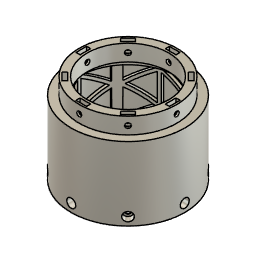
section_fuselage_30mm_ISO v15 (Autodesk Fusion 360 design; units mm, degrees)
Autodesk Fusion 360 part; units mm, degrees
note: some values were not read from the file. Set by a fixed rule: which face or edge a step refers to.
sketch "Esquisse1" plane through (0, 0, 0) normal (0, 1, 0) x (1, 0, 0)
  circle A0 centre (0, 0) radius 35
  circle A1 centre (0, 0) radius 30
  dimension "d1" = 70
  dimension "d2" = 60
  constraint coincident A0.centre A1.centre
  measures "d1" diameter of A0
  measures "d2" diameter of A1
extrude "Extrusion1" add sketch "Esquisse1" along normal mid plane 150 makes body 1
ref_plane "Plan de construction1" through (-30, 0, 0) normal (1, 0, 0) x (0, 1, 0)
sketch "Esquisse2" plane through (-30, 0, 0) normal (1, 0, 0) x (0, 0, -1)
  line L0 (-10, 75) -> (10, 75) construction
  line L1 (10, -75) -> (-10, -75) construction
  line L2 (0, 75) -> (0, -75) construction
  line L3 (0, 75) -> (0, 55) construction
  line L4 (0, 55) -> (0, 75) construction
  line L5 (0, 75) -> (17.3205, 65) construction
  line L6 (17.3205, 65) -> (0, 55) construction
  line L7 (0, 75) -> (-0.866, 75.5) construction
  line L8 (0, 75) -> (0, 76) construction
  line L9 (0.6, 54.2) -> (17.8202, 64.1338)
  line L10 (-0.494, 74.1306) -> (0, 75) construction
  line L11 (0, 75) -> (0.5, 75.866) construction
  line L12 (0.5, 75.866) -> (17.8205, 65.866)
  line L13 (15.4471, 65.0724) -> (1, 73.2816)
  line L14 (0, 73.8498) -> (-0.494, 74.1306)
  line L15 (1, 74.4227) -> (1, 75)
  line L16 (16.3207, 65.5772) -> (16.8202, 65.8658)
  line L17 (1, 56.7245) -> (1, 73.2816)
  line L18 (1, 56.7245) -> (15.4471, 65.0724)
  line L19 (-1, 56.7245) -> (-15.4471, 65.0724)
  line L20 (-1, 56.7245) -> (-1, 73.2816)
  line L21 (-15.4471, 65.0724) -> (-1, 73.2816)
  line L22 (-17.3205, 65) -> (0, 75) construction
  line L23 (0, 55) -> (-17.3205, 65) construction
  line L24 (-1, 74.4227) -> (-1, 75)
  line L25 (-1, 56.7245) -> (-1, 73.2816)
  line L26 (-16.3211, 66.5862) -> (-1.9882, 74.9932)
  line L27 (-16.327, 83.2717) -> (-16.3211, 66.5862)
  line L28 (-16.327, 83.2717) -> (-1.9882, 74.9932)
  circle A0 centre (-17.3205, 85) radius 1
  line L29 (16.327, 83.2717) -> (1.9882, 74.9932)
  line L30 (16.3211, 66.5862) -> (1.9882, 74.9932)
  line L31 (16.327, 83.2717) -> (16.3211, 66.5862)
  circle A1 centre (17.3205, 85) radius 1
  line L32 (-20.0336, 74.9932) -> (20, 74.9932)
  line L33 (0, 55) -> (-5, 55) construction
  line L34 (-1.9935, 55.0038) -> (-16.4465, 63.3414)
  line L35 (-16.4465, 63.3414) -> (-16.3323, 46.7252)
  line L36 (-1.9935, 55.0038) -> (-16.3323, 46.7252)
  line L37 (-0.9935, 53.2717) -> (-0.9994, 36.5862)
  line L38 (-0.9935, 53.2717) -> (-15.3323, 44.9932)
  line L39 (-0.9994, 36.5862) -> (-15.3323, 44.9932)
  line L40 (1.9935, 55.0038) -> (16.4465, 63.3414)
  line L41 (1.9935, 55.0038) -> (16.3323, 46.7252)
  line L42 (16.4465, 63.3414) -> (16.3323, 46.7252)
  line L43 (0.9935, 53.2717) -> (15.3323, 44.9932)
  line L44 (0.9994, 36.5862) -> (15.3323, 44.9932)
  line L45 (0.9935, 53.2717) -> (0.9994, 36.5862)
  line L46 (0, 35) -> (-15, 35) construction
  line L47 (-16.4465, 6.6586) -> (-16.3323, 23.2748)
  line L48 (-1.9935, 14.9962) -> (-16.4465, 6.6586)
  line L49 (-1, 13.2755) -> (-15.4471, 4.9276)
  line L50 (-15.4471, 4.9276) -> (-1, -3.2816)
  line L51 (-1, 13.2755) -> (-1, -3.2816)
  line L52 (15.4471, 4.9276) -> (1, -3.2816)
  line L53 (1, 13.2755) -> (1, -3.2816)
  line L54 (1, 13.2755) -> (15.4471, 4.9276)
  line L55 (1.9935, 14.9962) -> (16.4465, 6.6586)
  line L56 (16.4465, 6.6586) -> (16.3323, 23.2748)
  line L57 (1.9935, 14.9962) -> (16.3323, 23.2748)
  line L58 (0.9994, 33.4138) -> (15.3323, 25.0068)
  line L59 (0.9935, 16.7283) -> (15.3323, 25.0068)
  line L60 (0.9935, 16.7283) -> (0.9994, 33.4138)
  line L61 (-0.9994, 33.4138) -> (-15.3323, 25.0068)
  line L62 (-0.9935, 16.7283) -> (-15.3323, 25.0068)
  line L63 (-1.9935, 14.9962) -> (-16.3323, 23.2748)
  line L64 (-0.9935, 16.7283) -> (-0.9994, 33.4138)
  line L65 (0, -5) -> (-10, -5) construction
  line L66 (-1.8734, 35.0724) -> (-16.3205, 43.2816)
  line L67 (-16.3205, 26.7245) -> (-16.3205, 43.2816)
  line L68 (-16.3205, 26.7245) -> (-1.8734, 35.0724)
  line L69 (0, 35) -> (17.3205, 45) construction
  line L70 (1.8734, 35.0724) -> (16.3205, 43.2816)
  line L71 (16.3205, 26.7245) -> (16.3205, 43.2816)
  line L72 (16.3205, 26.7245) -> (1.8734, 35.0724)
  line L73 (0, -5) -> (-10, -5) construction
  line L74 (-15.4471, -14.9276) -> (-1, -6.7184)
  line L75 (-1, -23.2755) -> (-15.4471, -14.9276)
  line L76 (-1.9935, -24.9962) -> (-16.4465, -16.6586)
  line L77 (-1.9935, -24.9962) -> (-16.3323, -33.2748)
  line L78 (-16.4465, -16.6586) -> (-16.3323, -33.2748)
  line L79 (-0.9994, -43.4138) -> (-15.3323, -35.0068)
  line L80 (-0.9935, -26.7283) -> (-15.3323, -35.0068)
  line L81 (0.9935, -26.7283) -> (15.3323, -35.0068)
  line L82 (0.9994, -43.4138) -> (15.3323, -35.0068)
  line L83 (0.9935, -26.7283) -> (0.9994, -43.4138)
  line L84 (-0.9935, -26.7283) -> (-0.9994, -43.4138)
  line L85 (1.9935, -24.9962) -> (16.3323, -33.2748)
  line L86 (16.4465, -16.6586) -> (16.3323, -33.2748)
  line L87 (1.9935, -24.9962) -> (16.4465, -16.6586)
  line L88 (1, -23.2755) -> (15.4471, -14.9276)
  line L89 (1, -23.2755) -> (1, -6.7184)
  line L90 (-1, -23.2755) -> (-1, -6.7184)
  line L91 (15.4471, -14.9276) -> (1, -6.7184)
  line L92 (0, -45) -> (-15, -45) construction
  line L93 (-1.9935, -65.0038) -> (-16.3323, -56.7252)
  line L94 (1.9935, -65.0038) -> (16.3323, -56.7252)
  line L95 (-1, -66.7245) -> (-15.4471, -75.0724)
  circle A2 centre (0, -85) radius 1
  line L96 (0.9935, -63.2717) -> (15.3323, -54.9932)
  line L97 (0, -45) -> (-15, -45) construction
  line L98 (-0.9935, -63.2717) -> (-0.9994, -46.5862)
  line L99 (-0.9994, -46.5862) -> (-15.3323, -54.9932)
  line L100 (-16.4465, -73.3414) -> (-16.3323, -56.7252)
  line L101 (-1.9935, -65.0038) -> (-16.4465, -73.3414)
  line L102 (-0.9935, -63.2717) -> (-15.3323, -54.9932)
  line L103 (0.9994, -46.5862) -> (15.3323, -54.9932)
  circle A3 centre (0, -85) radius 1
  line L104 (0, -85) -> (-10, -85) construction
  line L105 (1, -66.7245) -> (15.4471, -75.0724)
  line L106 (-1, -66.7245) -> (-1, -83.2816)
  line L107 (0, -85) -> (-10, -85) construction
  line L108 (-15.4471, -75.0724) -> (-1, -83.2816)
  line L109 (16.4465, -73.3414) -> (16.3323, -56.7252)
  line L110 (1.9935, -65.0038) -> (16.4465, -73.3414)
  line L111 (15.4471, -75.0724) -> (1, -83.2816)
  line L112 (1, -66.7245) -> (1, -83.2816)
  line L113 (0.9935, -63.2717) -> (0.9994, -46.5862)
  line L114 (-20, -75) -> (25, -75)
  line L115 (-17.3205, 5) -> (0, -5) construction
  line L116 (0, -5) -> (17.3205, 5) construction
  line L117 (-17.3205, -35) -> (0, -45) construction
  line L118 (0, -45) -> (17.3205, -35) construction
  line L119 (-1.8734, -44.9276) -> (-16.3205, -36.7184)
  line L120 (-16.3205, -53.2755) -> (-16.3205, -36.7184)
  line L121 (-16.3205, -53.2755) -> (-1.8734, -44.9276)
  line L122 (16.3205, -53.2755) -> (1.8734, -44.9276)
  line L123 (16.3205, -53.2755) -> (16.3205, -36.7184)
  line L124 (1.8734, -44.9276) -> (16.3205, -36.7184)
  line L125 (-16.3211, 3.4138) -> (-1.9882, -4.9932)
  line L126 (-16.327, -13.2717) -> (-16.3211, 3.4138)
  line L127 (-16.327, -13.2717) -> (-1.9882, -4.9932)
  line L128 (16.327, -13.2717) -> (1.9882, -4.9932)
  line L129 (16.327, -13.2717) -> (16.3211, 3.4138)
  line L130 (16.3211, 3.4138) -> (1.9882, -4.9932)
  point P0 (0, -25)
  point P1 (0, -65)
  dimension "d7" = 20
  dimension "d9" = 20
  dimension "d10" = 60
  constraint horizontal L0
  constraint parallel L0 L1
  constraint midpoint L0 L2.start
  constraint midpoint L1 L2.end
  constraint perpendicular L1 L2
  constraint coincident L2 L3.end
  constraint coincident L0 L15.end
  constraint parallel L4 L8
  constraint perpendicular L7 L11
  constraint coincident L2 L14.start
  constraint collinear L13 L14
  constraint coincident L5 L15.start
  constraint coincident L5 L16.start
  constraint symmetric L3 L13.end L20.end
  constraint symmetric L3 L13.start L19.end
  constraint symmetric L3 L17.start L19.start
  constraint coincident L22 L24.start
  constraint symmetric L19.start L22 L27.start
  constraint symmetric L19.end L22 L26.start
  constraint symmetric L20.end L22 L26.end
  constraint symmetric L5 L13.end L29.end
  constraint symmetric L5 L13.start L30.start
  constraint symmetric L5 L17.start L29.start
  constraint parallel L0 L32
  constraint symmetric L13.end L23 L38.end
  constraint symmetric L13.start L23 L37.end
  constraint symmetric L17.start L23 L37.start
  constraint symmetric L19.start L23 L34.start
  constraint symmetric L19.end L23 L34.end
  constraint symmetric L20.end L23 L35.end
  constraint symmetric L6 L13.end L41.end
  constraint symmetric L6 L13.start L40.end
  constraint symmetric L6 L17.start L40.start
  constraint symmetric L2 L37.start L43.start
  constraint symmetric L2 L37.end L44.start
  constraint symmetric L2 L38.end L43.end
  constraint perpendicular L2 L46
  constraint symmetric L13.end L46 L52.end
  constraint symmetric L13.start L46 L52.start
  constraint symmetric L17.start L46 L53.start
  constraint symmetric L19.start L46 L49.start
  constraint symmetric L19.end L46 L49.end
  constraint symmetric L20.end L46 L50.end
  constraint symmetric L37.end L46 L61.start
  constraint symmetric L44.start L46 L58.start
  constraint symmetric L43.start L69 L71.start
  constraint symmetric L43.end L69 L70.end
  constraint symmetric L44.start L69 L70.start
  constraint symmetric L47.start L65 L76.end
  constraint symmetric L47.end L65 L77.end
  constraint symmetric L48.start L65 L76.start
  constraint symmetric L49.start L65 L75.start
  constraint symmetric L49.end L65 L74.start
  constraint symmetric L50.end L65 L74.end
  constraint symmetric L52.start L65 L88.end
  constraint symmetric L52.end L65 L89.end
  constraint symmetric L53.start L65 L88.start
  constraint symmetric L55.start L65 L85.start
  constraint symmetric L55.end L65 L86.start
  constraint symmetric L56.end L65 L85.end
  constraint symmetric L58.start L65 L82.start
  constraint symmetric L58.end L65 L81.end
  constraint symmetric L59.start L65 L81.start
  constraint symmetric L61.start L65 L79.start
  constraint symmetric L61.end L65 L79.end
  constraint symmetric L62.start L65 L80.start
  constraint symmetric L73.end L65 L65.end
  constraint symmetric L65.end L92 L104.end
  constraint symmetric P0 L92 P1
  constraint symmetric L74.start L92 L95.end
  constraint symmetric L74.end L92 L106.end
  constraint symmetric L75.start L92 L95.start
  constraint symmetric L76.start L92 L93.start
  constraint symmetric L76.end L92 L100.start
  constraint symmetric L77.end L92 L93.end
  constraint symmetric L79.start L92 L98.end
  constraint symmetric L79.end L92 L99.end
  constraint symmetric L80.start L92 L98.start
  constraint symmetric L81.start L92 L96.start
  constraint symmetric L81.end L92 L96.end
  constraint symmetric L82.start L92 L103.start
  constraint symmetric L85.start L92 L94.start
  constraint symmetric L85.end L92 L94.end
  constraint symmetric L86.start L92 L109.start
  constraint symmetric L88.start L92 L105.start
  constraint symmetric L88.end L92 L105.end
  constraint symmetric L89.end L92 L111.end
  constraint symmetric L97.start L92 L117.end
  constraint symmetric L97.end L92 L92.end
  constraint perpendicular L106 L114
  constraint symmetric L79.start L117 L119.start
  constraint symmetric L79.end L117 L119.end
  constraint symmetric L80.start L117 L120.start
  constraint symmetric L81.start L118 L122.start
  constraint symmetric L81.end L118 L123.end
  constraint symmetric L82.start L118 L122.end
  constraint symmetric L49.start L115 L126.start
  constraint symmetric L49.end L115 L125.start
  constraint symmetric L50.end L115 L125.end
  constraint symmetric L52.start L116 L129.end
  constraint symmetric L52.end L116 L128.end
  constraint symmetric L53.start L116 L128.start
  measures "d7" distance of L2.start L3.end
  measures "d9" distance of L2.start L5.end
  measures "d10" angle of L4 L5
emboss "Gravure en relief1" depth -2 profiles "Esquisse2" section 1 contours L9 L40 L41 L42 | L12 L31 L32 | L12 L30 L31 L32 | L13 L17 L18 | L19 L20 L21 L25 | L26 L27 L32 | L34 L35 L36 | L37 L38 L39 | L43 L44 L45 | L47 L48 L63 | L49 L50 L51 | L52 L53 L54 | L55 L56 L57 | L58 L59 L60 | L61 L62 L64 | L66 L67 L68 | L70 L71 L72 | L74 L75 L90 | L76 L77 L78 | L79 L80 L84 | L81 L82 L83 | L85 L86 L87 | L88 L89 L91 | L93 L100 L101 | L94 L109 L110 | L95 L106 L114 | L96 L103 L113 | L98 L99 L102 | L105 L112 L114 | L119 L120 L121 | L122 L123 L124 | L125 L126 L127 | L128 L129 L130 onto face at (29.9627, 50, 1.4954) on bodies 1 bodies 1
pattern_circular "Réseau C1" count 5 over 360 about axis through (0, 1.75, 0) along (0, 1, 0) of "Gravure en relief1"
extrude "Extrusion2" cut 1 faces at (33.0913, 75, 3.2292) along direction (0, -1, 0) blind 120 on bodies 1 bodies 1
sketch "Esquisse1 (2)" plane through (0, 0, 0) normal (0, 1, 0) x (1, 0, 0) in component "couplage_standard_femelle v11"
  circle A0 centre (0, 0) radius 35
  circle A1 centre (0, 0) radius 30
  dimension "d1_1" = 70
  dimension "d2_1" = 60
  constraint coincident A0.centre A1.centre
  constraint concentric A0 A1
  measures "d1_1" diameter of A0
  measures "d2_1" diameter of A1
extrude "Extrusion1'" add sketch "Esquisse1 (2)" along normal mid plane 10 separate body makes body 2 in component "couplage_standard_femelle v11"
ref_plane "Plan de construction1" through (35, 0, 0) normal (1, 0, 0) x (0, 1, 0) in component "couplage_standard_femelle v11"
ref_plane "Plan de construction2" through (-35, 0, 0) normal (1, 0, 0) x (0, 1, 0) in component "couplage_standard_femelle v11"
ref_plane "Plan de construction3" through (0, 0, 35) normal (0, 0, 1) x (1, 0, 0) in component "couplage_standard_femelle v11"
ref_plane "Plan de construction4" through (0, 0, -35) normal (0, 0, 1) x (1, 0, 0) in component "couplage_standard_femelle v11"
sketch "Esquisse2 (2)" plane through (35, 0, 0) normal (1, 0, 0) x (0, 0, -1) in component "couplage_standard_femelle v11"
  circle A0 centre (0, 0) radius 1.5
  circle A1 centre (0, 0) radius 2.25
  dimension "d9_1" = 3
  dimension "d10_1" = 4.5
  constraint coincident A0.centre A1.centre
  constraint concentric A0 A1
  measures "d9_1" diameter of A0
  measures "d10_1" diameter of A1
extrude "Extrusion2'" cut sketch "Esquisse2 (2)" against normal blind 70 contours A0 bodies 2 in component "couplage_standard_femelle v11"
extrude "Extrusion3" cut sketch "Esquisse2 (2)" against normal blind 3 bodies 2 in component "couplage_standard_femelle v11"
sketch "Esquisse3" plane through (-35, 0, 0) normal (1, 0, 0) x (0, 0, -1) in component "couplage_standard_femelle v11"
  circle A0 centre (0, 0) radius 2.25
  circle A1 centre (0, 0) radius 1.5
extrude "Extrusion4" cut sketch "Esquisse3" along normal blind 3 bodies 2 in component "couplage_standard_femelle v11"
sketch "Esquisse4" plane through (0, 0, 35) normal (0, 0, 1) x (1, 0, 0) in component "couplage_standard_femelle v11"
  circle A0 centre (0, 0) radius 1.5
  circle A1 centre (0, 0) radius 2.25
  dimension "d17_1" = 3
  dimension "d18_1" = 4.5
  constraint coincident A0.centre A1.centre
  measures "d17_1" diameter of A0
  measures "d18_1" diameter of A1
extrude "Extrusion5" cut sketch "Esquisse4" against normal blind 70 contours A0 bodies 2 in component "couplage_standard_femelle v11"
extrude "Extrusion6" cut sketch "Esquisse4" against normal blind 3 bodies 2 in component "couplage_standard_femelle v11"
sketch "Esquisse5" plane through (0, 0, -35) normal (0, 0, 1) x (1, 0, 0) in component "couplage_standard_femelle v11"
  circle A0 centre (0, 0) radius 1.5
  circle A1 centre (0, 0) radius 2.25
extrude "Extrusion7" cut sketch "Esquisse5" along normal blind 3 bodies 2 in component "couplage_standard_femelle v11"
move_body "Déplacer1" bodies 2 to x (0.707107, 0, 0.707107) y (0, 1, 0) z (-0.707107, 0, 0.707107) at (0, 0, 0) in component "couplage_standard_femelle v11"
ref_plane "Plan de construction5" through (35, 0, 0) normal (1, 0, 0) x (0, 1, 0) in component "couplage_standard_femelle v11"
ref_plane "Plan de construction6" through (-35, 0, 0) normal (1, 0, 0) x (0, 1, 0) in component "couplage_standard_femelle v11"
ref_plane "Plan de construction7" through (0, 0, 35) normal (0, 0, 1) x (1, 0, 0) in component "couplage_standard_femelle v11"
ref_plane "Plan de construction8" through (0, 0, -35) normal (0, 0, 1) x (1, 0, 0) in component "couplage_standard_femelle v11"
extrude "Extrusion8" cut sketch "Esquisse4" against normal blind 70 contours A0 bodies 2 in component "couplage_standard_femelle v11"
extrude "Extrusion9" cut sketch "Esquisse4" against normal blind 3 bodies 2 in component "couplage_standard_femelle v11"
sketch "Esquisse6" plane through (0, 0, -35) normal (0, 0, 1) x (1, 0, 0) in component "couplage_standard_femelle v11"
  circle A0 centre (0, 0) radius 2.25
  circle A1 centre (0, 0) radius 1.5
extrude "Extrusion10" cut sketch "Esquisse6" along normal blind 3 bodies 2 in component "couplage_standard_femelle v11"
sketch "Esquisse7" plane through (-35, 0, 0) normal (1, 0, 0) x (0, 0, -1) in component "couplage_standard_femelle v11"
  circle A0 centre (0, 0) radius 1.5
  circle A1 centre (0, 0) radius 2.25
  dimension "d35" = 3
  dimension "d36" = 4.5
  constraint coincident A0.centre A1.centre
  measures "d35" diameter of A0
  measures "d36" diameter of A1
extrude "Extrusion11" cut sketch "Esquisse7" along normal blind 70 contours A0 bodies 2 in component "couplage_standard_femelle v11"
extrude "Extrusion12" cut sketch "Esquisse7" along normal blind 3 bodies 2 in component "couplage_standard_femelle v11"
sketch "Esquisse8" plane through (35, 0, 0) normal (1, 0, 0) x (0, 0, -1) in component "couplage_standard_femelle v11"
  circle A0 centre (0, 0) radius 2.25
  circle A1 centre (0, 0) radius 1.5
extrude "Extrusion13" cut sketch "Esquisse8" against normal blind 3 bodies 2 in component "couplage_standard_femelle v11"
move_face "DécalerLesFaces1" offset -0.5 8 faces at (23.3345, 2.25, 23.3345) (33, 2.25, 0) (23.3345, 2.25, -23.3345) (0, 2.25, -33) (-23.3345, 2.25, -23.3345) (-33, 2.25, 0) (-23.3345, 2.25, 23.3345) (0, 2.25, 33) on bodies 2 in component "couplage_standard_femelle v11"
extrude "Extrusion14" cut 1 faces at (32, -0.2111, -2.3175) along direction (-1, 0, 0) blind 1 on bodies 2 bodies 2 in component "couplage_standard_femelle v11"
extrude "Extrusion15" cut 1 faces at (24.2661, -0.2111, -20.9887) along direction (-0.707107, 0, 0.707107) blind 1 on bodies 2 bodies 2 in component "couplage_standard_femelle v11"
extrude "Extrusion16" cut 1 faces at (2.3231, -0.1366, -32) along direction (0, 0, 1) blind 1 on bodies 2 bodies 2 in component "couplage_standard_femelle v11"
extrude "Extrusion17" cut 1 faces at (-20.9847, -0.1366, -24.2701) along direction (0.707107, 0, 0.707107) blind 1 on bodies 2 bodies 2 in component "couplage_standard_femelle v11"
extrude "Extrusion18" cut 1 faces at (-32, -0.2111, -2.3175) along direction (1, 0, 0) blind 1 on bodies 2 bodies 2 in component "couplage_standard_femelle v11"
extrude "Extrusion19" cut 1 faces at (-20.9887, -0.2111, 24.2661) along direction (0.707107, 0, -0.707107) blind 1 on bodies 2 bodies 2 in component "couplage_standard_femelle v11"
extrude "Extrusion20" cut 1 faces at (2.3231, -0.1366, 32) along direction (0, 0, -1) blind 1 on bodies 2 bodies 2 in component "couplage_standard_femelle v11"
extrude "Extrusion21" cut 1 faces at (24.2701, -0.1366, 20.9847) along direction (-0.707107, 0, -0.707107) blind 1 on bodies 2 bodies 2 in component "couplage_standard_femelle v11"
move_face "DécalerLesFaces2" offset -0.5 1 faces at (-5.7003, -0.0323, 29.4535) on bodies 2 in component "couplage_standard_femelle v11"
combine "Combiner1" operation add target body 1 tool bodies 2 body 2 seen with x (1, 0, 0) y (0, 1, 0) z (0, 0, 1) at (0, -80, 0)
sketch "Esquisse1 (3)" plane through (0, 0, 0) normal (0, 1, 0) x (1, 0, 0) in component "couplage_standard_male v8"
  circle A0 centre (0, 0) radius 30
  circle A1 centre (0, 0) radius 25
  dimension "d1_2" = 60
  constraint coincident A0.centre A1.centre
  constraint concentric A0 A1
  measures "d1_2" diameter of A0
extrude "Extrusion1''" add sketch "Esquisse1 (3)" along normal mid plane 10 separate body makes body 3 in component "couplage_standard_male v8"
sketch "Esquisse2 (3)" plane through (0, -5, 0) normal (0, -1, 0) x (1, 0, 0) in component "couplage_standard_male v8"
  circle A0 centre (0, 0) radius 25
  circle A1 centre (0, 0) radius 30
  circle A2 centre (0, 0) radius 35
  dimension "d4_2" = 70
  constraint coincident A0.centre A1.centre
  measures "d4_2" diameter of A2
extrude "Extrusion2''" add sketch "Esquisse2 (3)" along normal blind 5 contours A1 | A2 bodies 3 in component "couplage_standard_male v8"
ref_plane "Plan de construction1" through (30, 0, 0) normal (1, 0, 0) x (0, 1, 0) in component "couplage_standard_male v8"
ref_plane "Plan de construction2" through (-30, 0, 0) normal (1, 0, 0) x (0, 1, 0) in component "couplage_standard_male v8"
ref_plane "Plan de construction3" through (0, 0, 30) normal (0, 0, 1) x (1, 0, 0) in component "couplage_standard_male v8"
ref_plane "Plan de construction4" through (0, 0, -30) normal (0, 0, 1) x (1, 0, 0) in component "couplage_standard_male v8"
sketch "Esquisse3 (2)" plane through (30, 0, 0) normal (1, 0, 0) x (0, 0, -1) in component "couplage_standard_male v8"
  circle A0 centre (0, 0) radius 1.5
  dimension "d11_1" = 3
  constraint coincident A0.centre origin
  measures "d11_1" diameter of A0
extrude "Extrusion3'" cut sketch "Esquisse3 (2)" against normal blind 60 bodies 3 in component "couplage_standard_male v8"
sketch "Esquisse4 (2)" plane through (0, 0, -30) normal (0, 0, 1) x (1, 0, 0) in component "couplage_standard_male v8"
  circle A0 centre (0, 0) radius 1.5
  dimension "d14_1" = 3
  constraint coincident A0.centre origin
  measures "d14_1" diameter of A0
extrude "Extrusion4'" cut sketch "Esquisse4 (2)" along normal blind 60 bodies 3 in component "couplage_standard_male v8"
sketch "Esquisse5 (2)" plane through (0, 5, 0) normal (0, 1, 0) x (-1, 0, 0) in component "couplage_standard_male v8"
  circle A0 centre (0, 0) radius 25
  circle A1 centre (0, 0) radius 30
  line L0 (0, 30) -> (0, 25) construction
  line L1 (0, 27.5) -> (-5, 27.5) construction
  line L2 (0, 27.5) -> (5, 27.5) construction
  line L3 (0, 27.5) -> (0, 26.25)
  line L4 (0, 27.5) -> (0, 28.75)
  line L5 (0, 26.25) -> (3.25, 26.25)
  line L6 (0, 28.75) -> (3.25, 28.75)
  line L7 (3.25, 28.75) -> (3.25, 26.25)
  line L8 (0, 26.25) -> (-3.25, 26.25)
  line L9 (0, 28.75) -> (-3.25, 28.75)
  line L10 (-3.25, 28.75) -> (-3.25, 26.25)
  line L11 (-18.5616, 18.5616) -> (-16.2635, 20.8597)
  line L12 (-19.4454, 19.4454) -> (-18.5616, 18.5616)
  line L13 (-19.4454, 19.4454) -> (-20.3293, 20.3293)
  line L14 (-20.3293, 20.3293) -> (-18.0312, 22.6274)
  line L15 (-18.0312, 22.6274) -> (-16.2635, 20.8597)
  line L16 (-18.5616, 18.5616) -> (-20.8597, 16.2635)
  line L17 (-22.6274, 18.0312) -> (-20.8597, 16.2635)
  line L18 (-20.3293, 20.3293) -> (-22.6274, 18.0312)
  line L19 (-19.4454, 19.4454) -> (-22.981, 15.9099) construction
  line L20 (-19.4454, 19.4454) -> (-15.9099, 22.981) construction
  line L21 (-21.2132, 21.2132) -> (-17.6777, 17.6777) construction
  line L22 (-26.25, 0) -> (-26.25, 3.25)
  line L23 (-27.5, 0) -> (-26.25, 0)
  line L24 (-27.5, 0) -> (-28.75, 0)
  line L25 (-28.75, 0) -> (-28.75, 3.25)
  line L26 (-28.75, 3.25) -> (-26.25, 3.25)
  line L27 (-26.25, 0) -> (-26.25, -3.25)
  line L28 (-28.75, -3.25) -> (-26.25, -3.25)
  line L29 (-28.75, 0) -> (-28.75, -3.25)
  line L30 (-27.5, 0) -> (-27.5, -5) construction
  line L31 (-27.5, 0) -> (-27.5, 5) construction
  line L32 (-30, 0) -> (-25, 0) construction
  line L33 (-18.5616, -18.5616) -> (-20.8597, -16.2635)
  line L34 (-19.4454, -19.4454) -> (-18.5616, -18.5616)
  line L35 (-19.4454, -19.4454) -> (-20.3293, -20.3293)
  line L36 (-20.3293, -20.3293) -> (-22.6274, -18.0312)
  line L37 (-22.6274, -18.0312) -> (-20.8597, -16.2635)
  line L38 (-18.5616, -18.5616) -> (-16.2635, -20.8597)
  line L39 (-18.0312, -22.6274) -> (-16.2635, -20.8597)
  line L40 (-20.3293, -20.3293) -> (-18.0312, -22.6274)
  line L41 (-19.4454, -19.4454) -> (-15.9099, -22.981) construction
  line L42 (-19.4454, -19.4454) -> (-22.981, -15.9099) construction
  line L43 (-21.2132, -21.2132) -> (-17.6777, -17.6777) construction
  line L44 (0, -26.25) -> (-3.25, -26.25)
  line L45 (0, -27.5) -> (0, -26.25)
  line L46 (0, -27.5) -> (0, -28.75)
  line L47 (0, -28.75) -> (-3.25, -28.75)
  line L48 (-3.25, -28.75) -> (-3.25, -26.25)
  line L49 (0, -26.25) -> (3.25, -26.25)
  line L50 (3.25, -28.75) -> (3.25, -26.25)
  line L51 (0, -28.75) -> (3.25, -28.75)
  line L52 (0, -27.5) -> (5, -27.5) construction
  line L53 (0, -27.5) -> (-5, -27.5) construction
  line L54 (0, -30) -> (0, -25) construction
  line L55 (18.5616, -18.5616) -> (16.2635, -20.8597)
  line L56 (19.4454, -19.4454) -> (18.5616, -18.5616)
  line L57 (19.4454, -19.4454) -> (20.3293, -20.3293)
  line L58 (20.3293, -20.3293) -> (18.0312, -22.6274)
  line L59 (18.0312, -22.6274) -> (16.2635, -20.8597)
  line L60 (18.5616, -18.5616) -> (20.8597, -16.2635)
  line L61 (22.6274, -18.0312) -> (20.8597, -16.2635)
  line L62 (20.3293, -20.3293) -> (22.6274, -18.0312)
  line L63 (19.4454, -19.4454) -> (22.981, -15.9099) construction
  line L64 (19.4454, -19.4454) -> (15.9099, -22.981) construction
  line L65 (21.2132, -21.2132) -> (17.6777, -17.6777) construction
  line L66 (26.25, 0) -> (26.25, -3.25)
  line L67 (27.5, 0) -> (26.25, 0)
  line L68 (27.5, 0) -> (28.75, 0)
  line L69 (28.75, 0) -> (28.75, -3.25)
  line L70 (28.75, -3.25) -> (26.25, -3.25)
  line L71 (26.25, 0) -> (26.25, 3.25)
  line L72 (28.75, 3.25) -> (26.25, 3.25)
  line L73 (28.75, 0) -> (28.75, 3.25)
  line L74 (27.5, 0) -> (27.5, 5) construction
  line L75 (27.5, 0) -> (27.5, -5) construction
  line L76 (30, 0) -> (25, 0) construction
  line L77 (18.5616, 18.5616) -> (20.8597, 16.2635)
  line L78 (19.4454, 19.4454) -> (18.5616, 18.5616)
  line L79 (19.4454, 19.4454) -> (20.3293, 20.3293)
  line L80 (20.3293, 20.3293) -> (22.6274, 18.0312)
  line L81 (22.6274, 18.0312) -> (20.8597, 16.2635)
  line L82 (18.5616, 18.5616) -> (16.2635, 20.8597)
  line L83 (18.0312, 22.6274) -> (16.2635, 20.8597)
  line L84 (20.3293, 20.3293) -> (18.0312, 22.6274)
  line L85 (19.4454, 19.4454) -> (15.9099, 22.981) construction
  line L86 (19.4454, 19.4454) -> (22.981, 15.9099) construction
  line L87 (21.2132, 21.2132) -> (17.6777, 17.6777) construction
  dimension "d17_2" = 1.25
  dimension "d18_2" = 1.25
  dimension "d19_2" = 3.25
  dimension "d20_2" = 3.25
  dimension "d21_2" = 3.25
  dimension "d25_1" = 360
  constraint coincident A1 L0.start
  constraint coincident A0 L0.end
  constraint vertical L0
  constraint midpoint L0 L1.start
  constraint perpendicular L0 L1
  constraint perpendicular L0 L2
  constraint coincident L0 L3.end
  constraint perpendicular L1 L4
  constraint perpendicular L3 L5
  constraint perpendicular L4 L6
  constraint perpendicular L3 L8
  constraint perpendicular L0 L9
  constraint perpendicular L8 L10
  measures "d17_2" distance of L1.start L3.end
  measures "d18_2" distance of L1.start L4.end
  measures "d19_2" distance of L3.end L5.end
  measures "d20_2" distance of L4.end L6.end
  measures "d21_2" distance of L3.end L8.end
extrude "Extrusion6'" cut sketch "Esquisse5 (2)" against normal blind 8 contours L3 L4 L5 L6 L7 | L3 L4 L8 L9 L10 | L11 L12 L13 L14 L15 | L12 L13 L16 L17 L18 | L22 L23 L24 L25 L26 | L23 L24 L27 L28 L29 | L33 L34 L35 L36 L37 | L34 L35 L38 L39 L40 | L44 L45 L46 L47 L48 | L45 L46 L49 L50 L51 | L55 L56 L57 L58 L59 | L56 L57 L60 L61 L62 | L66 L67 L68 L69 L70 | L67 L68 L71 L72 L73 | L77 L78 L79 L80 L81 | L78 L79 L82 L83 L84 bodies 3 in component "couplage_standard_male v8"
move_body "Déplacer1'" bodies 3 to x (0.707107, 0, 0.707107) y (0, 1, 0) z (-0.707107, 0, 0.707107) at (0, 0, 0) in component "couplage_standard_male v8"
ref_plane "Plan de construction5" through (0, 0, -30) normal (0, 0, 1) x (1, 0, 0) in component "couplage_standard_male v8"
ref_plane "Plan de construction6" through (30, 0, 0) normal (1, 0, 0) x (0, 1, 0) in component "couplage_standard_male v8"
sketch "Esquisse6 (2)" plane through (30, 0, 0) normal (1, 0, 0) x (0, 0, -1) in component "couplage_standard_male v8"
  circle A0 centre (0, 0) radius 1.5
  dimension "d30_1" = 3
  constraint coincident A0.centre origin
  measures "d30_1" diameter of A0
sketch "Esquisse7 (2)" plane through (0, 0, -30) normal (0, 0, 1) x (1, 0, 0) in component "couplage_standard_male v8"
  circle A0 centre (0, 0) radius 1.5
  dimension "d31_1" = 3
  constraint coincident A0.centre origin
  measures "d31_1" diameter of A0
extrude "Extrusion7'" cut sketch "Esquisse6 (2)" against normal blind 60 bodies 3 in component "couplage_standard_male v8"
extrude "Extrusion8'" cut sketch "Esquisse7 (2)" along normal blind 60 bodies 3 in component "couplage_standard_male v8"
chamfer "Chanfrein1" distance 5 angle 45 1 edges at (-22.8739, -10, -10.0889) on bodies 3 in component "couplage_standard_male v8"
chamfer "Chanfrein1'" distance 0.5 angle 45 5 edges at (-30, -75, 0) (-9.2705, -75, 28.5317) (24.2705, -75, 17.6336) (24.2705, -75, -17.6336) (-9.2705, -75, -28.5317) on bodies 1
combine "Combiner3" operation add target body 1 tool bodies 3 body 3 seen with x (1, 0, 0) y (0, 1, 0) z (0, 0, 1) at (0, -35, 0)
move_body "Déplacer1''" bodies 1 to x (1, 0, 0) y (0, 1, 0) z (0, 0, 1) at (0, 60, 0)
component "couplage_standard_femelle v11" placed x (1, 0, 0) y (0, 1, 0) z (0, 0, 1) at (0, -80, 0)
component "couplage_standard_male v8" placed x (1, 0, 0) y (0, 1, 0) z (0, 0, 1) at (0, -35, 0)
equation "d17_2 = ( 2.5 / 2 ) * 1 mm"
equation "d18_2 = ( 2.5 / 2 ) * 1 mm"
equation "d19_2 = ( 6.5 / 2 ) * 1 mm"
equation "d20_2 = ( 6.5 / 2 ) * 1 mm"
equation "d21_2 = ( 6.5 / 2 ) * 1 mm"
named bodies: "section_isogrid_30mm"
